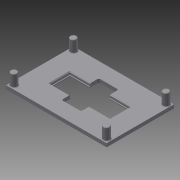
# Autodesk Inventor part: 1x3 slide SD stage insert
Saved by Autodesk Inventor 2013 (Build 170138000, 138)
## iProperties
Created: 2012-10-15
Part Number: 1x3 slide SD stage insert
Material: Generic
Document SubType Name: Modeling
Designer: kthorn
Density: 1 g/cm^3
Author: kthorn
Autodesk Inventor part; units mm, degrees
ref_plane "YZ Plane" through (0, 0, 0) normal (1, 0, 0) x (0, 1, 0)
ref_plane "XZ Plane" through (0, 0, 0) normal (0, 1, 0) x (-1, 0, 0)
ref_plane "XY Plane" through (0, 0, 0) normal (0, 0, 1) x (1, 0, 0)
sketch "Sketch1" plane through (0, 0, 0) normal (0, 0, 1) x (1, 0, 0)
  line L0 (-63.85, 42.75) -> (63.85, 42.75)
  line L1 (63.85, 42.75) -> (63.85, -42.75)
  line L2 (63.85, -42.75) -> (-63.85, -42.75)
  line L3 (-63.85, -42.75) -> (-63.85, 42.75)
  line L4 (-63.85, 42.75) -> (63.85, -42.75) construction
  line L5 (63.85, 42.75) -> (-63.85, -42.75) construction
  point P0 (0, 0)
  dimension "d0" = 127.7
  dimension "d1" = 85.5
  constraints: 12 end point, 2 midpoint, 2 parallel, 1 horizontal, 1 perpendicular
  measures "d0" distance of L1.end L2.end
  measures "d1" distance of L0.end L1.end
extrude "Extrusion1" add sketch "Sketch1" along normal blind 4.5
sketch "Sketch2" plane through (0, 0, 4.5) normal (0, 0, 1) x (1, 0, 0)
  line L0 (-38.25, 12.75) -> (38.25, 12.75)
  line L1 (38.25, 12.75) -> (38.25, -12.75)
  line L2 (38.25, -12.75) -> (-38.25, -12.75)
  line L3 (-38.25, -12.75) -> (-38.25, 12.75)
  line L4 (-38.25, 12.75) -> (38.25, -12.75) construction
  line L5 (38.25, 12.75) -> (-38.25, -12.75) construction
  point P0 (0, 0)
  dimension "d4" = 76.5
  dimension "d5" = 25.5
  constraints: 12 end point, 2 midpoint, 2 parallel, 1 horizontal, 1 perpendicular
  measures "d4" distance of L1.end L2.end
  measures "d5" distance of L0.end L1.end
extrude "Extrusion2" cut sketch "Sketch2" against normal blind 3.5
sketch "Sketch3" plane through (0, 0, 1) normal (0, 0, 1) x (1, 0, 0)
  line L0 (-38.25, 12.75) -> (38.25, 12.75) projected
  line L1 (38.25, 12.75) -> (38.25, -12.75) projected
  line L2 (-37.25, 11.75) -> (37.25, 11.75)
  line L3 (37.25, 11.75) -> (37.25, -11.75)
  line L4 (37.25, -11.75) -> (-37.25, -11.75)
  line L5 (-37.25, -11.75) -> (-37.25, 11.75)
  line L6 (-37.25, 11.75) -> (37.25, -11.75) construction
  line L7 (37.25, 11.75) -> (-37.25, -11.75) construction
  line L8 (0, 11.75) -> (0, 12.75) construction
  line L9 (37.25, 0) -> (38.25, 0) construction
  point P0 (0, 0)
  dimension "d8" = 1
  constraints: 16 end point, 6 midpoint, 2 parallel, 2 perpendicular, 1 horizontal
  measures "d8" distance of L8.start L8.end
extrude "Extrusion3" cut sketch "Sketch3" against normal through all
chamfer "Chamfer1" distance 1 angle 45 4 edges at (-38.25, 0, 4.5) (0, 12.75, 4.5) (38.25, 0, 4.5) (0, -12.75, 4.5)
sketch "Sketch4" plane through (0, 0, 4.5) normal (0, 0, 1) x (1, 0, 0)
  line L0 (63.85, 42.75) -> (-63.85, 42.75) projected
  circle A0 centre (-58.85, 37.75) radius 4
  line L1 (-63.85, 42.75) -> (-58.85, 42.75) construction
  line L2 (-58.85, 42.75) -> (-58.85, 37.75) construction
  line L3 (-63.85, 42.75) -> (-63.85, -42.75) projected
  line L4 (-63.85, -42.75) -> (63.85, -42.75) projected
  line L5 (63.85, -42.75) -> (63.85, 42.75) projected
  line L6 (0, 42.75) -> (0, -42.75) construction
  line L7 (-63.85, 0) -> (63.85, 0) construction
  circle A1 centre (58.85, 37.75) radius 4
  circle A2 centre (-58.85, -37.75) radius 4
  circle A3 centre (58.85, -37.75) radius 4
  point P0 (0, 0)
  dimension "d15" = 8
  dimension "d17" = 5
  constraints: 8 end point, 4 centre point, 4 midpoint, 3 symmetric about line, 2 perpendicular, 1 coincident, 1 point on line, 3 other
  measures "d15" diameter of A0
  measures "d17" distance of L1.end L2.end
extrude "Extrusion4" add sketch "Sketch4" along normal blind 15 contours A0 | A1 | A2 | A3
fillet "Fillet1" radius 1 8 edges at (-62.85, 37.75, 19.5) (-62.85, 37.75, 4.5) (-62.85, -37.75, 19.5) (-62.85, -37.75, 4.5) (54.85, 37.75, 19.5) (54.85, 37.75, 4.5) (54.85, -37.75, 19.5) (54.85, -37.75, 4.5)
sketch "Sketch5" plane through (0, 0, 4.5) normal (0, 0, 1) x (1, 0, 0)
  line L0 (39.25, 13.75) -> (-39.25, 13.75) projected
  line L1 (-12.5, 23.75) -> (12.5, 23.75)
  line L2 (12.5, 23.75) -> (12.5, -23.75)
  line L3 (12.5, -23.75) -> (-12.5, -23.75)
  line L4 (-12.5, -23.75) -> (-12.5, 23.75)
  line L5 (-12.5, 23.75) -> (12.5, -23.75) construction
  line L6 (12.5, 23.75) -> (-12.5, -23.75) construction
  line L7 (0, 23.75) -> (0, 13.75) construction
  point P0 (0, 0)
  dimension "d22" = 10
  dimension "d24" = 25
  constraints: 14 end point, 4 midpoint, 2 parallel, 1 horizontal, 1 perpendicular
  measures "d22" distance of L7.start L7.end
  measures "d24" distance of L1.start L1.end
extrude "Extrusion5" cut sketch "Sketch5" against normal through all
fillet "Fillet2" radius 2 4 edges at (-12.5, 23.75, 2.25) (12.5, 23.75, 2.25) (-12.5, -23.75, 2.25) (12.5, -23.75, 2.25)
body "Solid1"
